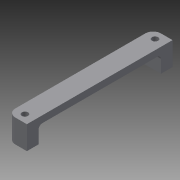
# Autodesk Inventor part: phone_clamp
Saved by Autodesk Inventor 2015 (Build 190159000, 159)
## iProperties
Created: 2015-12-01
Part Number: phone_clamp
Material: Generic
Document SubType Name: Modeling
Designer: jufranz
Density: 1 g/cm^3
Appearance: Default
Author: jufranz
Autodesk Inventor part; units mm, degrees
ref_plane "YZ Plane" through (0, 0, 0) normal (1, 0, 0) x (0, 1, 0)
ref_plane "XZ Plane" through (0, 0, 0) normal (0, 1, 0) x (-1, 0, 0)
ref_plane "XY Plane" through (0, 0, 0) normal (0, 0, 1) x (1, 0, 0)
sketch "Sketch1" plane through (0, 0, 0) normal (0, 1, 0) x (-1, 0, 0)
  line L0 (5, 37.5) -> (-5, 37.5)
  line L1 (-5, 37.5) -> (-5, -37.5)
  line L2 (-5, -37.5) -> (5, -37.5)
  line L3 (5, -37.5) -> (5, 37.5)
  point P0 (0, 0)
  point P1 (5, 0)
  point P2 (0, 37.5)
  dimension "d0" = 10
  dimension "d1" = 75
  constraints: 8 end point, 2 midpoint, 2 parallel, 1 horizontal, 1 horizontal alignment, 1 perpendicular, 1 vertical alignment
  measures "d0" distance of L0.start L0.end
  measures "d1" distance of L2.end L0.start
extrude "Extrusion1" add sketch "Sketch1" along normal blind 12
sketch "Sketch2" plane through (5, 0, 37.5) normal (1, 0, 0) x (0, 0, -1)
  line L0 (6, 0) -> (69, 0)
  line L1 (69, 0) -> (69, 6.5)
  line L2 (67, 8.5) -> (8, 8.5)
  line L3 (6, 6.5) -> (6, 0)
  line L4 (0, 0) -> (75, 0) projected
  arc A0 (8, 8.5) -> (6, 6.5) centre (8, 6.5) ccw
  arc A1 (69, 6.5) -> (67, 8.5) centre (67, 6.5) ccw
  point P0 (37.5, 0)
  point P1 (37.5, 0)
  dimension "d4" = 63
  dimension "d5" = 8.5
  dimension "d6" = 2
  constraints: 8 end point, 4 point on circle, 4 tangent, 2 centre point, 2 midpoint, 2 parallel, 1 equal radius, 1 horizontal, 1 perpendicular
  measures "d4" distance between parallel lines of L1 L3
  measures "d5" distance between parallel lines of L0 L2
  measures "d6" radius of A0
extrude "Extrusion2" cut sketch "Sketch2" against normal through all
sketch "Sketch3" plane through (0, 12, 0) normal (0, 1, 0) x (1, 0, 0)
  point P0 (0, 0)
  point P1 (0, 33.5)
  point P2 (0, -33.5)
  dimension "d9" = 67
  dimension "d10" = 33.5
  constraints: 2 vertical alignment
  measures "d9" distance of point (0, -33.5) point (0, 33.5)
  measures "d10" distance of point (0, 0) point (0, 33.5)
hole "Hole1" at (0, 12, -33.5) at (0, 12, 33.5) direction (0, -1, 0) diameter 3.2 end through all
fillet "Fillet1" radius 4 2 edges at (-5, 6, 37.5) (-5, 6, -37.5)
equation "\"d10\" = 0.5 * d9"
body "Solid1"
